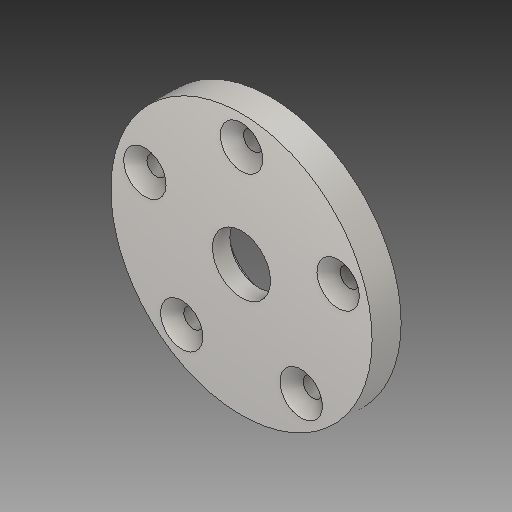
# Autodesk Inventor part: 342-08
Saved by Autodesk Inventor 2019 (Build 230136000, 136)
## iProperties
Company: Autodesk Inc.
Created: 2017-06-23
Part Number: 342-08
Material: Titanium
Document SubType Name: Modeling
Designer: Autodesk Inc.
Density: 4.51 g/cm^3
Appearance: Stainless - Brushed
Mass: 249.137 g
Surface Area: 164.02 cm^2
Volume: 55.2409 cm^3
Author: Inventor
Autodesk Inventor part; units mm, degrees
ref_plane "YZ Plane" through (0, 0, 0) normal (1, 0, 0) x (0, 1, 0)
ref_plane "XZ Plane" through (0, 0, 0) normal (0, 1, 0) x (-1, 0, 0)
ref_plane "XY Plane" through (0, 0, 0) normal (0, 0, 1) x (1, 0, 0)
sketch "Sketch1" plane through (0, 0, 0) normal (0, 0, 1) x (1, 0, 0)
  circle A0 centre (0, 0) radius 45
  circle A1 centre (0, 0) radius 10
  dimension "d0" = 90
  dimension "d1" = 20
  constraints: 2 centre point, 2 coincident
  measures "d0" diameter of A0
  measures "d1" diameter of A1
extrude "Extrusion1" add sketch "Sketch1" along normal blind 10
hole "Hole1" at (0, 0, 0) direction (0, 0, 1) diameter 30 depth 4
sketch "Sketch2" plane through (0, 0, 0) normal (0, 0, -1) x (-1, 0, 0)
  circle A0 centre (0, 35) radius 3.6674
  point P0 (0, 0)
  dimension "d15" = 35
  constraints: 1 centre point
  measures "d15" distance of A0.centre point (0, 0)
hole "Hole2" at (0, 35, 0) direction (0, 0, 1) diameter 6.6 end through all counterbore diameter 12 counterbore depth 2
chamfer "Chamfer1" distance 4 angle 45 1 edges at (0, 31.7, 10)
pattern_circular "Circular Pattern1" count 5 over 360 about axis through (0, 0, 0) along (0, 0, 1) of "Hole2", "Chamfer1"
body "Solid1"
